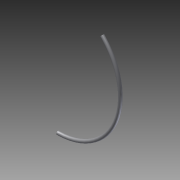
# Autodesk Inventor part: 8 ball arch
Saved by Autodesk Inventor 2012 (Build 160160000, 160)
## iProperties
Created: 2013-09-05
Part Number: 8 ball arch
Material: Default
Document SubType Name: Modeling
Designer: Bryce
Density: 1 g/cm^3
Author: Bryce
Autodesk Inventor part; units mm, degrees
ref_plane "YZ Plane" through (0, 0, 0) normal (1, 0, 0) x (0, 1, 0)
ref_plane "XZ Plane" through (0, 0, 0) normal (0, 1, 0) x (-1, 0, 0)
ref_plane "XY Plane" through (0, 0, 0) normal (0, 0, 1) x (1, 0, 0)
sketch "Sketch1" plane through (0, 0, 0) normal (0, 0, 1) x (1, 0, 0)
  arc A0 (0, -177.8) -> (125.7236, 125.7236) centre (0, 0) ccw
  line L0 (0, 0) -> (0, -177.8) construction
  line L1 (0, 0) -> (125.7236, 125.7236) construction
  dimension "d0" = 177.8
  dimension "d1" = 135
  constraints: 4 end point, 2 point on circle, 1 centre point, 1 coincident, 1 vertical
  measures "d0" radius of A0
  measures "d1" angle of L0 L1
sketch "Sketch2" plane through (0, 0, 0) normal (1, 0, 0) x (0, 1, 0)
  circle A0 centre (-177.8, 0) radius 4.7625
  circle A1 centre (-177.8, 0) radius 3.9688
  point P0 (0, 0)
  dimension "d2" = 9.525
  dimension "d3" = 7.9375
  constraints: 2 centre point, 2 coincident
  measures "d2" diameter of A0
  measures "d3" diameter of A1
sweep "Sweep1" add profiles "Sketch2" path "Sketch1"
body "Solid1"
